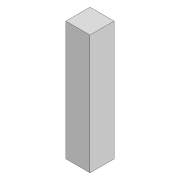
# Autodesk Inventor part: Aluminium_extrusion
Saved by Autodesk Inventor 2022 (Build 260153000, 153)
## iProperties
Created: 2022-07-04
Part Number: Aluminium_extrusion
Material: Generic
Document SubType Name: Modeling
Designer: dell
Density: 1 g/cm^3
Appearance: Default
Author: dell
Autodesk Inventor part; units mm, degrees
ref_plane "YZ Plane" through (0, 0, 0) normal (1, 0, 0) x (0, 1, 0)
ref_plane "XZ Plane" through (0, 0, 0) normal (0, 1, 0) x (-1, 0, 0)
ref_plane "XY Plane" through (0, 0, 0) normal (0, 0, 1) x (1, 0, 0)
sketch "Sketch1" plane through (0, 0, 0) normal (0, 1, 0) x (-1, 0, 0)
  line L0 (10.1, 10.1) -> (-10.1, 10.1)
  line L1 (-10.1, 10.1) -> (-10.1, -10.1)
  line L2 (-10.1, -10.1) -> (10.1, -10.1)
  line L3 (10.1, -10.1) -> (10.1, 10.1)
  line L4 (10.1, 10.1) -> (-10.1, -10.1) construction
  line L5 (-10.1, 10.1) -> (10.1, -10.1) construction
  point P0 (0, 0)
  dimension "d0" = 20.2
  dimension "d1" = 20.2
  constraints: 12 end point, 2 midpoint, 2 parallel, 1 horizontal, 1 perpendicular
  measures "d0" distance of L1.end L2.end
  measures "d1" distance of L0.end L1.end
extrude "Extrusion1" add sketch "Sketch1" along normal blind 100
body "Solid1"
